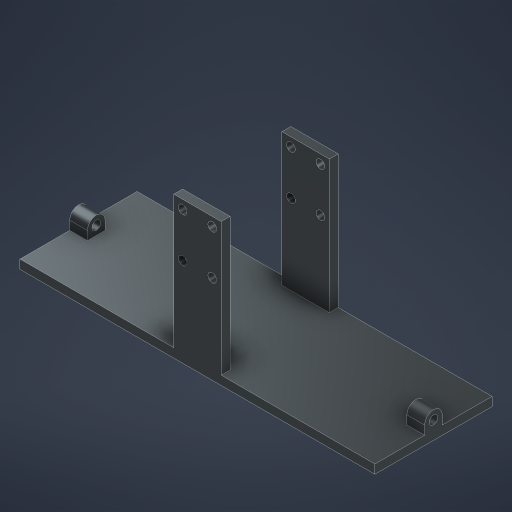
# Autodesk Inventor part: FP V2 Mounting Plate
Saved by Autodesk Inventor 2023.6 (Build 276521000, 521)
## iProperties
Created: 2026-02-15
Part Number: FP V2 Mounting Plate
Material: Aluminum 6061
Document SubType Name: Modeling
Designer: user
Density: 2.7 g/cm^3
Appearance: Iron Gray
Author: user
Autodesk Inventor part; units mm, degrees
ref_plane "YZ Plane" through (0, 0, 0) normal (1, 0, 0) x (0, 1, 0)
sketch "Sketch1" plane through (0, 0, 0) normal (0, 0, 1) x (1, 0, 0)
  line L0 (100, -2.5) -> (-100, -2.5)
  line L1 (-100, -2.5) -> (-100, 2.5)
  line L2 (-100, 2.5) -> (100, 2.5)
  line L3 (100, 2.5) -> (100, -2.5)
  line L4 (100, -2.5) -> (-100, 2.5) construction
  line L5 (-100, -2.5) -> (100, 2.5) construction
  point P0 (0, 0)
  dimension "d0" = 200
  dimension "d1" = 5
  constraints: 12 end point, 2 midpoint, 2 parallel, 1 horizontal, 1 perpendicular
  measures "d0" distance between parallel lines of L3 L1
  measures "d1" distance between parallel lines of L0 L2
extrude "Extrusion1" add sketch "Sketch1" along normal blind 66
sketch "Sketch2" plane through (0, 0, 0) normal (0, 0, -1) x (-1, 0, 0)
  line L0 (-8.35, 72.5) -> (8.35, 72.5)
  line L1 (8.35, 72.5) -> (8.35, 47.5)
  line L2 (8.35, 47.5) -> (-8.35, 47.5)
  line L3 (-8.35, 47.5) -> (-8.35, 72.5)
  line L4 (-8.35, 72.5) -> (8.35, 47.5) construction
  line L5 (8.35, 72.5) -> (-8.35, 47.5) construction
  line L6 (-13.35, -2.5) -> (13.35, -2.5)
  line L7 (13.35, -2.5) -> (13.35, 77.5)
  line L8 (13.35, 77.5) -> (-13.35, 77.5)
  line L9 (-13.35, 77.5) -> (-13.35, -2.5)
  line L10 (-13.35, -2.5) -> (13.35, 77.5) construction
  line L11 (13.35, -2.5) -> (-13.35, 77.5) construction
  circle A0 centre (-8.35, 47.5) radius 2.5
  circle A1 centre (8.35, 47.5) radius 2.5
  circle A2 centre (8.35, 72.5) radius 2.5
  circle A3 centre (-8.35, 72.5) radius 2.5
  line L12 (-100, 2.5) -> (100, 2.5) projected
  line L13 (100, -2.5) -> (-100, -2.5) projected
  point P0 (0, -2.5)
  dimension "d4" = 25
  dimension "d5" = 16.7
  dimension "d6" = 5
  dimension "d7" = 5
  dimension "d8" = 5
  dimension "d11" = 5
  dimension "d12" = 5
  dimension "d13" = 5
  dimension "d14" = 5
  dimension "d33" = 50
  constraints: 24 end point, 4 centre point, 4 coincident, 4 parallel, 2 horizontal, 2 midpoint, 2 perpendicular
  measures "d4" distance between parallel lines of L2 L0
  measures "d5" distance between parallel lines of L1 L3
  measures "d6" distance between parallel lines of L8 L0
  measures "d7" distance between parallel lines of L9 L3
  measures "d8" distance between parallel lines of L7 L1
  measures "d11" diameter of A0
  measures "d12" diameter of A1
  measures "d13" diameter of A2
  measures "d14" diameter of A3
  measures "d33" distance between parallel lines of L6 L2
extrude "Extrusion3" cut sketch "Sketch2" along normal blind 5 contours L3 A3 L0 | L0 A3 L3 | A2 L1 L0 | L0 L1 A2 | A0 L2 L3 | L3 L2 A0 | A1 L2 L1 | L1 L2 A1
sketch "Sketch3" plane through (-100, 2.5, 66) normal (0, 1, 0) x (1, 0, 0)
  line L0 (200, 66) -> (0, 66) projected
  line L1 (0, 66) -> (0, 0) projected
  line L2 (200, 0) -> (0, 0) projected
  line L3 (200, 66) -> (200, 0) projected
  line L4 (0, 66) -> (0, 0) projected
  line L5 (200, 66) -> (200, 0) projected
  line L6 (100, 33) -> (100, 66)
  line L7 (100, 33) -> (100, 0)
  line L8 (0, 0) -> (200, 0) projected
  line L9 (100, 33) -> (200, 33)
  circle A0 centre (100, 33) radius 4
  circle A1 centre (150, 33) radius 4
  line L10 (100, 33) -> (200, 33)
  line L11 (200, 66) -> (200, 0) projected
  line L12 (150, 33) -> (100, 33)
  dimension "d17" = 8
  dimension "d18" = 8
  dimension "d23" = 50
  constraints: 10 end point, 4 midpoint, 2 centre point, 1 perpendicular
  measures "d17" diameter of A0
  measures "d18" diameter of A1
  measures "d23" distance of L6.start A1.centre
sketch "Sketch5" plane through (-100, -2.5, 0) normal (-1, 0, 0) x (0, 0, 1)
  circle A0 centre (33, 10) radius 2.5
  circle A1 centre (33, 10) radius 5
  line L0 (0, 5) -> (0, 20) projected
  line L1 (0, 5) -> (66, 5)
  line L2 (0, 5) -> (66, 5) projected
  line L3 (28, 5) -> (28, 10)
  line L4 (38, 5) -> (38, 10)
  point P0 (0, 2.5)
  point P1 (33, 5)
  point P2 (28, 5)
  point P3 (38, 5)
  dimension "d29" = 5
  dimension "d30" = 10
  constraints: 6 end point, 3 point on circle, 2 centre point, 2 point on line, 2 tangent, 1 coincident, 1 horizontal, 1 midpoint, 1 perpendicular
  measures "d29" diameter of A0
  measures "d30" diameter of A1
extrude "Extrusion7" add sketch "Sketch5" against normal blind 10
ref_plane "Work Plane2" through (0, -2.5, 0) normal (-1, 0, 0) x (0, 0, 1)
mirror "Mirror2" about plane through (0, -2.5, 0) normal (-1, 0, 0) of "Extrusion7"
extrude "Extrusion8" add sketch "Sketch2" against normal blind 5 contours L0 A2 L1 A1 L2 A0 L3 A3 | L9 L12 L7 L6 | L9 L8 L7 L12
ref_plane "Work Plane3" through (0, 0, 33) normal (0, 0, -1) x (-1, 0, 0)
mirror "Mirror3" about plane through (0, 0, 33) normal (0, 0, -1) of "Extrusion8"
body "Solid1"
